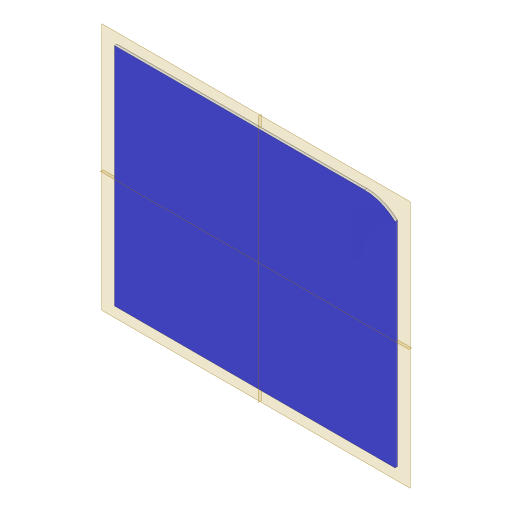
# Autodesk Inventor part: Боковая часть корпуса
Saved by Autodesk Inventor 2023.2 (Build 272271030, 271C)
## iProperties
Created: 2025-04-24
Part Number: Боковая часть корпуса
Material: Типовые
Document SubType Name: Modeling
Designer: Коноваленко
Density: 1 g/cm^3
Appearance: По умолчанию
Author: Коноваленко
Autodesk Inventor part; units mm, degrees
sketch "Эскиз1" plane through (0, 0, 0) normal (0, 0, 1) x (1, 0, 0)
  line L0 (223.6111, 170.1389) -> (223.6111, -179.8611)
  line L1 (223.6111, -179.8611) -> (-236.3889, -179.8611)
  line L2 (-236.3889, -179.8611) -> (-236.3889, 190.1389)
  line L3 (-236.3889, 190.1389) -> (223.6111, -179.8611) construction
  line L4 (223.6111, 170.1389) -> (-236.3889, -179.8611) construction
  line L5 (-328.7741, 0) -> (317.9221, 0) construction
  line L6 (0, 269.9164) -> (0, -254.824) construction
  line L7 (-236.3889, 190.1389) -> (173.6111, 190.1389)
  arc A0 (223.6111, 170.1389) -> (173.6111, 190.1389) centre (173.6111, 117.6389) ccw
  point P0 (0, 0)
  point P1 (0, 0)
  dimension "d2" = 370
  dimension "d3" = 350
  dimension "d4" = 460
  dimension "d13" = 72.5
  constraints: 12 end point, 4 point on line, 3 perpendicular, 2 point on circle, 1 centre point, 1 horizontal, 1 tangent
  measures "d2" distance of L1.end L2.end
  measures "d3" distance of L0.start L0.end
  measures "d4" distance of L0.end L1.end
  measures "d13" radius of A0
extrude "Выдавливание1" add sketch "Эскиз1" along normal mid plane 4
